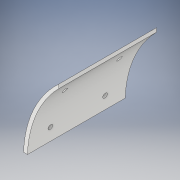
# Autodesk Inventor part: SJ009
Saved by Autodesk Inventor 2017 SP1 (Build 210196100, 196)
## iProperties
Created: 2017-06-10
Part Number: SJ009
Material: ABS Plastic
Document SubType Name: Modeling
Designer: Zach
Density: 1.06 g/cm^3
Appearance: CR White
Author: Zach
Autodesk Inventor part; units mm, degrees
ref_plane "YZ Plane" through (0, 0, 0) normal (1, 0, 0) x (0, 1, 0)
ref_plane "XZ Plane" through (0, 0, 0) normal (0, 1, 0) x (-1, 0, 0)
ref_plane "XY Plane" through (0, 0, 0) normal (0, 0, 1) x (1, 0, 0)
sketch "Sketch1" plane through (0, 0, 0) normal (0, 0, 1) x (1, 0, 0)
  arc A0 (45, 98) -> (0, 0) centre (139.9137, -4.9145) ccw
  line L0 (45, 98) -> (45, 93)
  line L1 (0, 0) -> (5, 0)
  arc A1 (45, 93) -> (5, 0) centre (144.908, -5.0734) ccw
  dimension "d0" = 140
  dimension "d1" = 98
  dimension "d3" = 45
  dimension "d4" = 5
  dimension "d5" = 5
  dimension "d6" = 140
  constraints: 4 end point, 4 point on circle, 2 centre point, 1 horizontal, 1 vertical
  measures "d0" radius of A0
  measures "d1" vertical distance of L1.start L0.start
  measures "d3" horizontal distance of L1.start L0.start
  measures "d4" distance of L0.start L0.end
  measures "d5" distance of L1.start L1.end
  measures "d6" radius of A1
extrude "Extrusion1" add sketch "Sketch1" along normal blind 125
sketch "Sketch2" plane through (0, 0, 0) normal (1, 0, 0) x (0, 1, 0)
  circle A0 centre (67.5, 27.5) radius 3
  circle A1 centre (17.5, 27.5) radius 3
  line L0 (98, 0) -> (98, 125) projected
  circle A2 centre (67.5, 97.5) radius 3
  circle A3 centre (17.5, 97.5) radius 3
  point P0 (0, 0)
  dimension "d9" = 6
  dimension "d10" = 6
  dimension "d11" = 27.5
  dimension "d12" = 50
  dimension "d13" = 30.5
  dimension "d14" = 6
  dimension "d15" = 6
  dimension "d16" = 70
  constraints: 4 centre point, 2 horizontal alignment, 2 vertical alignment
  measures "d9" diameter of A0
  measures "d10" diameter of A1
  measures "d11" vertical distance of point (0, 0) A0.centre
  measures "d12" distance of A1.centre A0.centre
  measures "d13" distance from line of A0.centre L0
  measures "d14" diameter of A2
  measures "d15" diameter of A3
  measures "d16" distance of A2.centre A0.centre
extrude "Extrusion2" cut sketch "Sketch2" along normal through all
body "Solid1"
